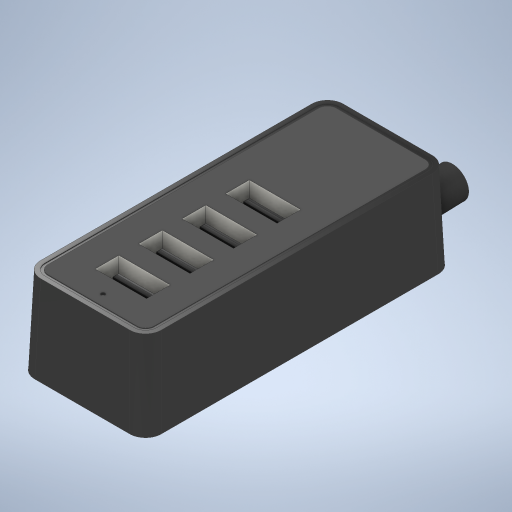
# Autodesk Inventor part: USB hub
Saved by Autodesk Inventor 2024.1 (Build 281209000, 209)
## iProperties
Created: 2025-04-13
Part Number: USB hub
Material: Generic
Document SubType Name: Modeling
Designer: User
Density: 1 g/cm^3
Appearance: Default
Author: User
Autodesk Inventor part; units mm, degrees
ref_plane "YZ Plane" through (0, 0, 0) normal (1, 0, 0) x (0, 1, 0)
ref_plane "XZ Plane" through (0, 0, 0) normal (0, 1, 0) x (-1, 0, 0)
ref_plane "XY Plane" through (0, 0, 0) normal (0, 0, 1) x (1, 0, 0)
sketch "Sketch1" plane through (0, 0, 0) normal (0, 1, 0) x (-1, 0, 0)
  line L0 (0, 0) -> (32, 0)
  line L1 (32, 0) -> (32, -78)
  line L2 (32, -78) -> (0, -78)
  line L3 (0, -78) -> (0, 0)
  dimension "d0" = 32
  dimension "d1" = 78
  constraints: 8 end point, 2 parallel, 1 horizontal, 1 perpendicular
  measures "d0" distance of L1.end L2.end
  measures "d1" distance of L0.end L1.end
extrude "Extrusion1" add sketch "Sketch1" along normal blind 22
chamfer "Chamfer2" distance 0.75 distance2 22 1 edges at (0, 22, -39) measured on face at (-21.3333, 22, -52)
chamfer "Chamfer3" distance 0.75 distance2 22 1 edges at (-16.3749, 22, 0) measured on face at (-21.5833, 22, -52)
chamfer "Chamfer4" distance 0.75 distance2 22 1 edges at (-32, 22, -39.3749) measured on face at (-21.5833, 22, -52.25)
chamfer "Chamfer5" distance 0.75 distance2 22 1 edges at (-16, 22, -78) measured on face at (-10.9166, 22, -26.4999)
sketch "Sketch2" plane through (0, 22, 0) normal (0, 1, 0) x (1, 0, 0)
  line L0 (-22.5, 9.75) -> (-9.5, 9.75)
  line L1 (-9.5, 9.75) -> (-9.5, 15.75)
  line L2 (-9.5, 15.75) -> (-22.5, 15.75)
  line L3 (-22.5, 15.75) -> (-22.5, 9.75)
  line L4 (-22.5, 20.75) -> (-9.5, 20.75)
  line L5 (-9.5, 20.75) -> (-9.5, 26.75)
  line L6 (-9.5, 26.75) -> (-22.5, 26.75)
  line L7 (-22.5, 26.75) -> (-22.5, 20.75)
  line L8 (-22.5, 31.75) -> (-9.5, 31.75)
  line L9 (-9.5, 31.75) -> (-9.5, 37.75)
  line L10 (-9.5, 37.75) -> (-22.5, 37.75)
  line L11 (-22.5, 37.75) -> (-22.5, 31.75)
  line L12 (-22.5, 42.75) -> (-9.5, 42.75)
  line L13 (-9.5, 42.75) -> (-9.5, 48.75)
  line L14 (-9.5, 48.75) -> (-22.5, 48.75)
  line L15 (-22.5, 48.75) -> (-22.5, 42.75)
  point P0 (0, 0)
  dimension "d19" = 13
  dimension "d20" = 6
  dimension "d21" = 13
  dimension "d22" = 6
  dimension "d23" = 13
  dimension "d24" = 6
  dimension "d25" = 13
  dimension "d26" = 6
  constraints: 32 end point, 8 parallel, 4 horizontal, 4 perpendicular, 2 point on line
  measures "d19" distance of L2.end L1.end
  measures "d20" distance of L1.end L0.end
  measures "d21" distance of L6.end L5.end
  measures "d22" distance of L5.end L4.end
  measures "d23" distance of L10.end L9.end
  measures "d24" distance of L9.end L8.end
  measures "d25" distance of L14.end L13.end
  measures "d26" distance of L13.end L12.end
extrude "Extrusion2" cut sketch "Sketch2" against normal blind 10
sketch "Sketch3" plane through (0, 12, 0) normal (0, 1, 0) x (1, 0, 0)
  line L0 (-21, 12.75) -> (-11, 12.75)
  line L1 (-11, 12.75) -> (-11, 14.25)
  line L2 (-11, 14.25) -> (-21, 14.25)
  line L3 (-21, 14.25) -> (-21, 12.75)
  line L4 (-21, 23.75) -> (-11, 23.75)
  line L5 (-11, 23.75) -> (-11, 25.25)
  line L6 (-11, 25.25) -> (-21, 25.25)
  line L7 (-21, 25.25) -> (-21, 23.75)
  line L8 (-21, 34.75) -> (-11, 34.75)
  line L9 (-11, 34.75) -> (-11, 36.25)
  line L10 (-11, 36.25) -> (-21, 36.25)
  line L11 (-21, 36.25) -> (-21, 34.75)
  line L12 (-21, 45.75) -> (-11, 45.75)
  line L13 (-11, 45.75) -> (-11, 47.25)
  line L14 (-11, 47.25) -> (-21, 47.25)
  line L15 (-21, 47.25) -> (-21, 45.75)
  point P0 (0, 0)
  dimension "d29" = 10
  dimension "d30" = 1.5
  dimension "d31" = 1.5
  dimension "d32" = 10
  dimension "d33" = 1.5
  dimension "d34" = 10
  dimension "d35" = 1.5
  constraints: 32 end point, 8 parallel, 4 horizontal, 4 perpendicular, 4 point on line
  measures "d29" distance of L2.end L1.end
  measures "d30" distance of L1.end L0.end
  measures "d31" distance of L5.end L4.end
  measures "d32" distance of L10.end L9.end
  measures "d33" distance of L9.end L8.end
  measures "d34" distance of L14.end L13.end
  measures "d35" distance of L13.end L12.end
extrude "Extrusion3" add sketch "Sketch3" along normal blind 8
sketch "Sketch4" plane through (0, 22, 0) normal (0, 1, 0) x (1, 0, 0)
  circle A0 centre (-16, 5.25) radius 0.5
  point P0 (0, 0)
  dimension "d38" = 1
  constraints: 1 centre point
  measures "d38" diameter of A0
extrude "Extrusion4" cut sketch "Sketch4" against normal blind 0.5
chamfer "Chamfer6" distance 0.5 angle 45 16 edges at (-16, 20, -12.75) (-11, 20, -13.5) (-16, 20, -14.25) (-21, 20, -13.5) (-21, 20, -24.5) (-16, 20, -23.75) (-11, 20, -24.5) (-16, 20, -25.25) (-21, 20, -35.5) (-16, 20, -34.75) (-16, 20, -36.25) (-11, 20, -35.5) (-21, 20, -46.5) (-16, 20, -45.75) (-16, 20, -47.25) (-11, 20, -46.5)
sketch "Sketch5" plane through (0, 22, 0) normal (0, 1, 0) x (1, 0, 0)
  line L0 (-31.25, 0.75) -> (-31.25, 77.25) projected
  line L1 (-0.75, 77.25) -> (-0.75, 0.75) projected
  line L2 (-31.25, 0.75) -> (-0.75, 0.75)
  line L3 (-0.75, 0.75) -> (-0.75, 77.25)
  line L4 (-0.75, 77.25) -> (-31.25, 77.25)
  line L5 (-31.25, 77.25) -> (-31.25, 0.75)
  line L6 (-30.15, 76.15) -> (-1.85, 76.15)
  line L7 (-1.85, 76.15) -> (-1.85, 1.85)
  line L8 (-1.85, 1.85) -> (-30.15, 1.85)
  line L9 (-30.15, 1.85) -> (-30.15, 76.15)
  line L10 (-2.55, 75.45) -> (-29.45, 75.45)
  line L11 (-29.45, 75.45) -> (-29.45, 2.55)
  line L12 (-29.45, 2.55) -> (-2.55, 2.55)
  line L13 (-2.55, 2.55) -> (-2.55, 75.45)
  point P0 (0, 0)
  dimension "d44" = 1.1
  dimension "d45" = 0.7
  constraints: 24 end point, 6 parallel, 3 perpendicular, 1 horizontal, 6 other
  measures "d44" distance between parallel lines of L4 L6
  measures "d45" distance between parallel lines of L6 L10
extrude "Extrusion5" cut sketch "Sketch5" against normal blind 0.2 contours L6 L7 L8 L9
fillet "Fillet1" radius 2.2 4 edges at (-29.45, 21.9, -2.55) (-2.55, 21.9, -2.55) (-2.55, 21.9, -75.45) (-29.45, 21.9, -75.45)
fillet "Fillet2" radius 2.9 4 edges at (-30.15, 21.9, -76.15) (-30.15, 21.9, -1.85) (-1.85, 21.9, -1.85) (-1.85, 21.9, -76.15)
fillet "Fillet3" radius 4 4 edges at (-0.375, 11, -77.6251) (-31.6251, 11.0001, -77.6251) (-31.6251, 11.0001, -0.3749) (-0.3749, 11, -0.3749)
sketch "Sketch6" plane through (-3.9977, 0, -78) normal (0, 0.0340711, -0.9994194) x (-1, 0, 0)
  circle A0 centre (6, 8) radius 4
  point P0 (-3.9977, 2.6575)
  dimension "d51" = 8
  constraints: 1 centre point
  measures "d51" diameter of A0
extrude "Extrusion6" add sketch "Sketch6" along normal blind 10
body "Solid1"
